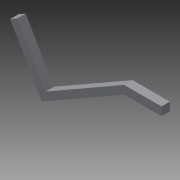
# Autodesk Inventor part: bar 2
Saved by Autodesk Inventor 2013 (Build 170138000, 138)
## iProperties
Created: 2013-03-02
Part Number: bar 2
Material: Generic
Document SubType Name: Modeling
Designer: Arpan
Density: 1 g/cm^3
Author: Arpan
Autodesk Inventor part; units mm, degrees
ref_plane "YZ Plane" through (0, 0, 0) normal (1, 0, 0) x (0, 1, 0)
ref_plane "XZ Plane" through (0, 0, 0) normal (0, 1, 0) x (-1, 0, 0)
ref_plane "XY Plane" through (0, 0, 0) normal (0, 0, 1) x (1, 0, 0)
sketch "Sketch1" plane through (0, 0, 0) normal (0, 0, 1) x (1, 0, 0)
  line L0 (0, 25.4) -> (0, 0)
  line L1 (-113.1604, 25.4) -> (-351.652, -111.264)
  line L2 (-351.652, -111.264) -> (-415.4102, 0)
  line L3 (-113.1604, 0) -> (-362.733, -143.0138)
  line L4 (-362.733, -143.0138) -> (-444.6849, 0)
  line L5 (-113.1604, 0) -> (0, 0)
  line L6 (-113.1604, 25.4) -> (0, 25.4)
  line L7 (0, 25.4) -> (0, 0)
  line L8 (0, 0) -> (-113.1604, 0)
  line L9 (0, 25.4) -> (-113.1604, 25.4)
  line L10 (-444.6849, 0) -> (-459.24, 25.4)
  line L11 (-459.24, 25.4) -> (-437.2019, 38.0286)
  line L12 (-437.2019, 38.0286) -> (-415.4102, 0)
  dimension "d0" = 25.4
  dimension "d1" = 25.4
  dimension "d2" = 25.4
  constraints: 26 end point, 4 collinear, 3 perpendicular
  measures "d0" distance of L3.start L1.start
  measures "d1" distance between parallel lines of L4 L2
  measures "d2" distance of L10.end L11.end
extrude "Extrusion1" add sketch "Sketch1" along normal blind 25.4
body "Solid1"
